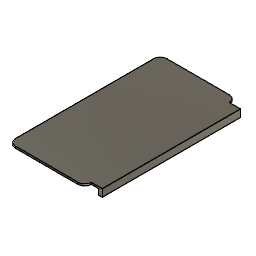
topBoard (Autodesk Fusion 360 design; units mm, degrees)
Autodesk Fusion 360 part; units mm, degrees
sketch "Sketch1" plane through (0, 0, 0) normal (0, 0, 1) x (1, 0, 0)
  line L0 (-50.8, 101.6) -> (50.8, 101.6)
  line L1 (50.8, 101.6) -> (50.8, -101.6)
  line L2 (50.8, -101.6) -> (-50.8, -101.6)
  line L3 (-50.8, -101.6) -> (-50.8, 101.6)
  line L4 (-50.8, 101.6) -> (50.8, -101.6) construction
  line L5 (50.8, 101.6) -> (-50.8, -101.6) construction
  dimension "d1" = 101.6
  dimension "d2" = 203.2
  constraint horizontal L0
  constraint vertical L1
  constraint horizontal L2
  constraint vertical L3
  constraint coincident origin L5
  constraint midpoint origin L4
  measures "d1" distance of L0.start L0.end
  measures "d2" distance of L0.start L2.end
extrude "Extrude1" add sketch "Sketch1" along normal blind 2.54
fillet "Fillet1" radius 8.89 4 edges at (-50.8, -101.6, 1.27) (50.8, -101.6, 1.27) (50.8, 101.6, 1.27) (-50.8, 101.6, 1.27)
extrude "Extrude4" add 1 faces at (50.8, 30.9033, 0.8467) along direction (1, 0, 0) blind 10
sketch "Sketch3" plane through (0, 0, 2.54) normal (0, 0, 1) x (-1, 0, 0)
  arc A0 (41.91, -101.6) -> (50.8, -92.71) centre (41.91, -92.71) ccw
  line L0 (50.8, -92.71) -> (50.8, 92.71)
  arc A1 (50.8, 92.71) -> (41.91, 101.6) centre (41.91, 92.71) ccw
  line L1 (41.91, 101.6) -> (-41.91, 101.6)
  arc A2 (-41.91, 101.6) -> (-50.8, 92.71) centre (-41.91, 92.71) ccw
  line L2 (-50.8, 92.71) -> (-60.8, 92.71)
  line L3 (-60.8, 92.71) -> (-60.8, -92.71)
  line L4 (-60.8, -92.71) -> (-50.8, -92.71)
  arc A3 (-50.8, -92.71) -> (-41.91, -101.6) centre (-41.91, -92.71) ccw
  line L5 (-41.91, -101.6) -> (41.91, -101.6)
  line L6 (-60.8, -92.71) -> (-65.8, -92.71)
  line L7 (-65.8, -92.71) -> (-65.8, 92.71)
  line L8 (-65.8, 92.71) -> (-60.8, 92.71)
  line L9 (-60.8, 92.71) -> (-60.8, -92.71)
  dimension "d28" = 5
  constraint horizontal L6
  constraint vertical L7
  constraint horizontal L8
  constraint vertical L9
  constraint coincident L3.end L4.start
  constraint horizontal L2.end L7.end
  measures "d28" distance of L3.end L6.end
extrude "Extrude5" add sketch "Sketch3" against normal blind 10 contours L3 L6 L7 L8 L9
sketch "Sketch4" plane through (0, 0, 0) normal (0, 0, -1) x (1, 0, 0)
  arc A0 (-50.8, -92.71) -> (-41.91, -101.6) centre (-41.91, -92.71) ccw
  line L0 (-41.91, -101.6) -> (41.91, -101.6)
  arc A1 (41.91, -101.6) -> (50.8, -92.71) centre (41.91, -92.71) ccw
  line L1 (50.8, -92.71) -> (60.8, -92.71)
  line L2 (60.8, -92.71) -> (60.8, 92.71)
  line L3 (60.8, 92.71) -> (50.8, 92.71)
  arc A2 (50.8, 92.71) -> (41.91, 101.6) centre (41.91, 92.71) ccw
  line L4 (41.91, 101.6) -> (-41.91, 101.6)
  arc A3 (-41.91, 101.6) -> (-50.8, 92.71) centre (-41.91, 92.71) ccw
  line L5 (-50.8, 92.71) -> (-50.8, -92.71)
  line L6 (50.8, -92.71) -> (50.8, 92.71) construction
  line L7 (-41.91, 92.71) -> (41.4111, 92.71)
  line L8 (41.4111, 92.71) -> (41.4111, -92.21)
  line L9 (41.4111, -92.21) -> (-41.91, -92.21)
  line L10 (-41.91, -92.21) -> (-41.91, 92.71)
  line L11 (-41.91, 92.71) -> (41.4111, -92.21) construction
  line L12 (41.4111, 92.71) -> (-41.91, -92.21) construction
  point P0 (-0.2495, 0.25)
  dimension "d32" = 184.92
  dimension "d36" = 83.3211
  constraint coincident A1.end L1.start
  constraint coincident L3.end A2.start
  constraint horizontal L7
  constraint vertical L8
  constraint horizontal L9
  constraint vertical L10
  constraint coincident A3.centre L7.start
  constraint midpoint L11 P0
  measures "d32" distance of L7.end L8.end
  measures "d36" distance of L8.end L9.end
extrude "Extrude6" add sketch "Sketch4" along normal blind 5 contours L7 L8 L9 L10
equation "d32 = 185.42 mm - 0.5 mm"
equation "d36 = 83.82109398 mm - 0.5 mm"
